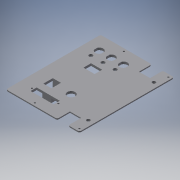
# Autodesk Inventor part: vrch2
Saved by Autodesk Inventor 2016 (Build 200138000, 138)
## iProperties
Created: 2015-11-06
Part Number: vrch2
Material: Generic
Document SubType Name: Modeling
Designer: Jufo
Density: 1 g/cm^3
Appearance: Default
Author: Jufo
Autodesk Inventor part; units mm, degrees
ref_plane "YZ Plane" through (0, 0, 0) normal (1, 0, 0) x (0, 1, 0)
ref_plane "XZ Plane" through (0, 0, 0) normal (0, 1, 0) x (-1, 0, 0)
ref_plane "XY Plane" through (0, 0, 0) normal (0, 0, 1) x (1, 0, 0)
sketch "Sketch1" plane through (0, 0, 0) normal (0, 1, 0) x (-1, 0, 0)
  line L0 (8.278, -23.2242) -> (24.278, -23.2242)
  line L1 (24.278, -23.2242) -> (24.278, 3.7758)
  line L2 (24.278, 3.7758) -> (48.278, 3.7758)
  line L3 (48.278, 3.7758) -> (48.278, -23.2242)
  line L4 (48.278, -23.2242) -> (88.278, -23.2242)
  line L5 (48.278, -23.2242) -> (136.1936, -23.2242)
  line L6 (136.1936, -23.2242) -> (136.1936, 142.7758)
  line L7 (136.1936, 142.7758) -> (48.278, 142.7758)
  line L8 (48.278, 142.7758) -> (48.278, 115.7758)
  line L9 (48.278, 115.7758) -> (24.278, 115.7758)
  line L10 (24.278, 115.7758) -> (24.278, 142.7758)
  line L11 (24.278, 142.7758) -> (24.278, 115.7758)
  line L12 (8.278, 142.7758) -> (24.278, 142.7758)
  line L13 (24.278, 142.7758) -> (8.278, 142.7758)
  line L14 (8.278, 142.7758) -> (8.278, -23.2242)
  line L15 (24.278, 3.7758) -> (24.278, -23.2242)
  circle A0 centre (11.278, -20.2242) radius 1.5
  circle A1 centre (11.278, -20.2242) radius 1.5
  circle A2 centre (11.278, 139.7758) radius 1.5
  circle A3 centre (11.278, 139.7758) radius 1.5
  circle A4 centre (91.278, -20.2242) radius 1.5
  circle A5 centre (91.278, -20.2242) radius 1.5
  circle A6 centre (91.278, 139.7758) radius 1.5
  circle A7 centre (91.278, 139.7758) radius 1.5
  line L16 (133.1936, 141.7758) -> (49.278, 141.7758)
  line L17 (49.278, 141.7758) -> (49.278, 114.7758)
  line L18 (49.278, 114.7758) -> (23.278, 114.7758)
  line L19 (23.278, 114.7758) -> (23.278, 141.7758)
  line L20 (8.278, 59.7758) -> (68.278, 59.7758)
  line L21 (133.1936, 141.7758) -> (133.1936, 59.7758)
  line L22 (23.278, 141.7758) -> (9.278, 141.7758)
  line L23 (9.278, 141.7758) -> (9.278, 59.7758)
  line L24 (133.1936, -22.2242) -> (49.278, -22.2242)
  line L25 (49.278, -22.2242) -> (49.278, 4.7758)
  line L26 (49.278, 4.7758) -> (23.278, 4.7758)
  line L27 (23.278, 4.7758) -> (23.278, -22.2242)
  line L28 (133.1936, -22.2242) -> (133.1936, 59.7758)
  line L29 (23.278, -22.2242) -> (9.278, -22.2242)
  line L30 (9.278, -22.2242) -> (9.278, 59.7758)
  point P0 (0, 0)
  point P1 (0, 0)
  dimension "d0" = 24
  dimension "d1" = 16
  dimension "d2" = 87.9156
  dimension "d3" = 166
  dimension "d4" = 3
  dimension "d5" = 27
  dimension "d6" = 1
  dimension "d8" = 1
  dimension "d9" = 1
  dimension "d10" = 1
  dimension "d11" = 1
  constraints: 62 end point, 13 perpendicular, 8 centre point, 6 symmetric about line, 5 point on line, 4 coincident, 3 horizontal, 2 parallel, 1 midpoint, 1 vertical
  measures "d0" distance of L8.end L9.end
  measures "d1" distance of L10.end L12.start
  measures "d2" distance of L6.end L7.end
  measures "d3" distance of L5.end L6.end
  measures "d4" distance between parallel lines of L6 L21
  measures "d5" distance of L7.end L8.end
  measures "d6" distance between parallel lines of L8 L17
  measures "d8" distance between parallel lines of L18 L9
  measures "d9" distance between parallel lines of L19 L10
  measures "d10" distance between parallel lines of L12 L22
  measures "d11" distance between parallel lines of L14 L23
extrude "Extrusion1" add sketch "Sketch1" along normal blind 2 contours L21 L28 L24 L25 L26 L27 L29 L30 L23 L22 L19 L18 L17 L16
sketch "Sketch2" plane through (0, 2, 0) normal (0, 1, 0) x (1, 0, 0)
  line L0 (-6.278, 25.2242) -> (-26.278, 25.2242)
  line L1 (-26.278, 25.2242) -> (-26.278, 2.2242)
  line L2 (-26.278, 2.2242) -> (-46.278, 2.2242)
  line L3 (-46.278, 2.2242) -> (-46.278, 25.2242)
  line L4 (-46.278, 25.2242) -> (-138.2936, 25.2242)
  line L5 (-133.1936, 22.2242) -> (-133.1936, -141.7758) projected
  line L6 (-133.1936, -59.7758) -> (-63.3349, -59.7758)
  line L7 (-138.2936, 25.2242) -> (-138.2936, -59.7758)
  line L8 (-6.278, 25.2242) -> (-6.278, -59.7758)
  line L9 (-9.278, -141.7758) -> (-9.278, 22.2242) projected
  line L10 (-9.278, 22.2242) -> (-23.278, 22.2242) projected
  line L11 (-23.278, 22.2242) -> (-23.278, -4.7758) projected
  line L12 (-23.278, -4.7758) -> (-49.278, -4.7758) projected
  line L13 (-49.278, -4.7758) -> (-49.278, 22.2242) projected
  line L14 (-49.278, 22.2242) -> (-133.1936, 22.2242) projected
  line L15 (-6.278, -144.7758) -> (-26.278, -144.7758)
  line L16 (-26.278, -144.7758) -> (-26.278, -121.7758)
  line L17 (-26.278, -121.7758) -> (-46.278, -121.7758)
  line L18 (-46.278, -121.7758) -> (-46.278, -144.7758)
  line L19 (-46.278, -144.7758) -> (-138.2936, -144.7758)
  line L20 (-6.278, -144.7758) -> (-6.278, -59.7758)
  line L21 (-138.2936, 25.2242) -> (-138.2936, -144.7758)
  circle A0 centre (-91.278, 20.2242) radius 1.5 projected
  circle A1 centre (-91.278, 20.2242) radius 1.5
  circle A2 centre (-91.278, -139.7758) radius 1.5 projected
  circle A3 centre (-91.278, -139.7758) radius 1.5
  circle A4 centre (-11.278, -139.7758) radius 1.5 projected
  circle A5 centre (-11.278, -139.7758) radius 1.5
  circle A6 centre (-11.278, 20.2242) radius 1.5
  point P0 (0, 0)
  dimension "d14" = 3
  dimension "d15" = 3
  dimension "d16" = 3
  dimension "d17" = 7
  dimension "d18" = 3
  dimension "d19" = 3
  dimension "d130" = 5.1
  constraints: 30 end point, 6 symmetric about line, 5 point on line, 4 centre point, 4 perpendicular, 3 coincident, 2 horizontal, 1 concentric, 1 midpoint, 1 parallel, 1 vertical
  measures "d14" distance between parallel lines of L8 L9
  measures "d15" distance between parallel lines of L0 L10
  measures "d16" distance between parallel lines of L1 L11
  measures "d17" distance between parallel lines of L12 L2
  measures "d18" distance between parallel lines of L13 L3
  measures "d19" distance between parallel lines of L4 L14
  measures "d130" distance between parallel lines of L5 L21
extrude "Extrusion2" add sketch "Sketch2" along normal blind 2
sketch "Sketch9" plane through (0, 4, 0) normal (0, 1, 0) x (1, 0, 0)
  line L0 (-26.278, -121.7758) -> (-6.278, -121.7758)
  line L1 (-6.278, -144.7758) -> (-6.278, 25.2242) projected
  line L2 (-26.278, 2.2242) -> (-6.278, 2.2242)
  line L3 (-16.278, -121.7758) -> (-16.278, -118.7758)
  circle A0 centre (-16.278, -118.7758) radius 3
  line L4 (-16.278, 2.2242) -> (-16.278, -0.7758)
  circle A1 centre (-16.278, -0.7758) radius 3
  line L5 (-102.439, -41.2758) -> (-82.439, -41.2758)
  line L6 (-82.439, -41.2758) -> (-82.439, -27.7758)
  line L7 (-82.439, -27.7758) -> (-102.439, -27.7758)
  line L8 (-102.439, -27.7758) -> (-102.439, -41.2758)
  line L9 (-26.278, 2.2242) -> (-46.278, 2.2242) projected
  line L10 (-26.278, 25.2242) -> (-26.278, 2.2242) projected
  line L11 (-113.628, -102.2758) -> (-99.128, -102.2758)
  line L12 (-99.128, -102.2758) -> (-99.128, -85.2758)
  line L13 (-99.128, -85.2758) -> (-113.628, -85.2758)
  line L14 (-113.628, -85.2758) -> (-113.628, -102.2758)
  circle A2 centre (-72.128, -93.7758) radius 7
  circle A3 centre (-114.678, -0.7758) radius 7
  circle A4 centre (-92.878, -0.7758) radius 7
  circle A5 centre (-71.078, -0.7758) radius 7
  line L15 (-121.6758, -0.6001) -> (-121.6758, -0.6001)
  line L16 (-99.8758, -0.9515) -> (-99.8758, -0.6001)
  circle A6 centre (-114.678, -15.7758) radius 3.25
  circle A7 centre (-92.878, -15.7758) radius 3.25
  circle A8 centre (-71.078, -15.7758) radius 3.25
  line L17 (-46.278, 25.2242) -> (-138.2936, 25.2242) projected
  line L18 (-49.278, -4.7758) -> (-49.278, 22.2242) projected
  line L19 (-138.2936, 25.2242) -> (-138.2936, -144.7758) projected
  line L20 (-113.628, -125.2758) -> (-72.128, -125.2758)
  line L21 (-72.128, -125.2758) -> (-72.128, -114.2758)
  line L22 (-72.128, -114.2758) -> (-113.628, -114.2758)
  line L23 (-113.628, -114.2758) -> (-113.628, -125.2758)
  line L24 (-46.278, -121.7758) -> (-26.278, -121.7758) projected
  line L25 (-113.628, -119.7758) -> (-116.628, -119.7758)
  circle A9 centre (-116.628, -119.7758) radius 1.5
  line L26 (-72.128, -119.7758) -> (-69.128, -119.7758)
  circle A10 centre (-69.128, -119.7758) radius 1.5
  line L27 (-99.0879, -4.0066) -> (-99.0879, 2.455)
  line L28 (-120.8879, -4.0066) -> (-120.8879, 2.455)
  line L29 (-77.2879, -4.0066) -> (-77.2879, 2.455)
  line L30 (-46.278, -144.7758) -> (-46.278, -121.7758) projected
  line L31 (-64.8682, 2.455) -> (-64.8682, -4.0066)
  line L32 (-86.6682, 2.455) -> (-86.6682, -4.0066)
  line L33 (-108.4682, 2.455) -> (-108.4682, -4.0066)
  arc A11 (-108.4682, -4.0066) -> (-108.4682, 2.455) centre (-114.678, -0.7758) ccw
  point P0 (0, 0)
  dimension "d62" = 3
  dimension "d63" = 6
  dimension "d64" = 3
  dimension "d65" = 13.5
  dimension "d66" = 20
  dimension "d67" = 30
  dimension "d69" = 20
  dimension "d70" = 17
  dimension "d71" = 14.5
  dimension "d72" = 14
  dimension "d75" = 14
  dimension "d76" = 14
  dimension "d77" = 14
  dimension "d78" = 21.8
  dimension "d79" = 21.8
  dimension "d80" = 6.5
  dimension "d81" = 6.5
  dimension "d82" = 6.5
  dimension "d83" = 15
  dimension "d84" = 15
  dimension "d85" = 15
  dimension "d89" = 21.8
  dimension "d90" = 21.8
  dimension "d92" = 21.8
  dimension "d93" = 21.8
  dimension "d97" = 11
  dimension "d98" = 41.5
  dimension "d99" = 7.5
  dimension "d100" = 3
  dimension "d101" = 3
  dimension "d102" = 3
  dimension "d103" = 3
  dimension "d106" = 25.85
  dimension "d108" = 0
  dimension "d109" = 20.5
  constraints: 52 end point, 18 point on circle, 12 centre point, 10 parallel, 7 vertical, 6 horizontal, 4 coincident, 4 midpoint, 3 perpendicular, 2 point on line, 1 concentric, 1 tangent
  measures "d62" distance of L3.start L3.end
  measures "d63" diameter of A0
  measures "d64" distance of L4.start L4.end
  measures "d65" distance of L5.end L6.end
  measures "d66" distance of L6.end L7.end
  measures "d67" distance between parallel lines of L9 L7
  measures "d69" distance between parallel lines of L1 L10
  measures "d70" distance of L11.end L12.end
  measures "d71" distance of L12.end L13.end
  measures "d72" diameter of A2
  measures "d75" diameter of A3
  measures "d76" diameter of A4
  measures "d77" diameter of A5
  measures "d78" distance of A4.centre A3.centre
  measures "d79" distance of A5.centre A4.centre
  measures "d80" diameter of A6
  measures "d81" diameter of A7
  measures "d82" diameter of A8
  measures "d83" distance of A6.centre A3.centre
  measures "d84" distance of A4.centre A7.centre
  measures "d85" distance of A5.centre A8.centre
  measures "d89" distance of A7.centre A8.centre
  measures "d90" distance of A7.centre A6.centre
  measures "d92" distance from line of L18 A8.centre
  measures "d93" distance from line of L18 A5.centre
  measures "d97" distance of L20.end L21.end
  measures "d98" distance of L21.end L22.end
  measures "d99" distance between parallel lines of L22 L24
  measures "d100" distance of L25.start L25.end
  measures "d101" diameter of A9
  measures "d102" distance of L26.start L26.end
  measures "d103" diameter of A10
  measures "d106" distance between parallel lines of L30 L21
  measures "d108" distance between parallel lines of L23 L14
  measures "d109" distance from line of A2.centre L22
extrude "Extrusion8" cut sketch "Sketch9" against normal blind 15 contours A0 | A1 | L8 L7 L6 L5 | L14 L13 L12 L11 | A2 | L33 A3 L28 | L32 A4 L27 | L31 A5 L29 | A6 | A7 | A8 | L23 L22 L21 L20 | A9 | A10
fillet "Fillet1" radius 3 8 edges at (-46.278, 3, -25.2242) (-26.278, 3, -25.2242) (-6.278, 3, -25.2242) (-6.278, 3, 144.7758) (-46.278, 3, 144.7758) (-26.278, 3, 144.7758) (-138.2936, 3, -25.2242) (-138.2936, 3, 144.7758)
sketch "Sketch10" plane through (0, 0, 0) normal (0, -1, 0) x (1, 0, 0)
  line L0 (-113.628, 85.2758) -> (-113.628, 83.2758)
  line L1 (-113.628, 83.2758) -> (-97.128, 83.2758)
  line L2 (-97.128, 83.2758) -> (-97.128, 104.2758)
  line L3 (-97.128, 104.2758) -> (-113.628, 104.2758)
  line L4 (-113.628, 104.2758) -> (-113.628, 102.2758)
  line L5 (-99.128, 102.2758) -> (-99.128, 85.2758) projected
  line L6 (-113.628, 102.2758) -> (-99.128, 102.2758) projected
  line L7 (-113.628, 85.2758) -> (-99.128, 85.2758)
  line L8 (-99.128, 85.2758) -> (-99.128, 102.2758)
  line L9 (-99.128, 102.2758) -> (-113.628, 102.2758)
  point P0 (0, 0)
  dimension "d112" = 2
  dimension "d113" = 2
  dimension "d114" = 2
  constraints: 16 end point, 5 perpendicular, 1 collinear, 1 horizontal, 1 point on line, 1 vertical
  measures "d112" distance of L0.start L0.end
  measures "d113" distance between parallel lines of L2 L5
  measures "d114" distance between parallel lines of L3 L6
extrude "Extrusion9" add sketch "Sketch10" along normal blind 17
sketch "Sketch11" plane through (0, 0, 0) normal (0, -1, 0) x (1, 0, 0)
  circle A0 centre (-72.128, 93.7758) radius 7 projected
  line L0 (-69.8349, 79.8078) -> (-67.8349, 79.8078)
  line L1 (-67.8349, 79.8078) -> (-67.8349, 84.7028)
  line L2 (-67.8349, 84.7028) -> (-69.8349, 84.7028)
  line L3 (-71.4349, 84.7028) -> (-71.4349, 79.8078)
  line L4 (-71.4349, 79.8078) -> (-73.4349, 79.8078)
  line L5 (-73.4349, 79.8078) -> (-73.4349, 84.7028)
  line L6 (-73.4349, 84.7028) -> (-71.4349, 84.7028)
  line L7 (-69.8349, 84.7028) -> (-69.8349, 79.8078)
  line L8 (-70.6349, 85.8044) -> (-70.6349, 78.1264)
  point P0 (0, 0)
  dimension "d117" = 2
  dimension "d118" = 2
  dimension "d120" = 0.8
  dimension "d121" = 0.8
  constraints: 18 end point, 5 perpendicular, 4 point on line, 2 vertical, 1 horizontal
  measures "d117" distance of L1.end L2.end
  measures "d118" distance of L5.end L3.start
  measures "d120" distance between parallel lines of L7 L8
  measures "d121" distance between parallel lines of L8 L3
extrude "Extrusion10" add sketch "Sketch11" along normal blind 8 contours L7 L2 L1 L0 | L3 L4 L5 L6
sketch "Sketch12" plane through (-67.8349, 0, 84.7028) normal (1, 0, 0) x (0, 0, -1)
  circle A0 centre (1.695, -6.5) radius 1
  line L0 (4.895, 0) -> (4.895, -8) projected
  line L1 (4.895, -8) -> (0, -8) projected
  point P0 (84.7028, 0)
  point P1 (0, 0)
  dimension "d124" = 2
  dimension "d126" = 3.2
  dimension "d127" = 1.5
  constraints: 1 centre point
  measures "d124" diameter of A0
  measures "d126" distance from line of L0 A0.centre
  measures "d127" distance from line of L1 A0.centre
extrude "Extrusion11" cut sketch "Sketch12" against normal blind 8
sketch "Sketch15" plane through (0, 2, 0) normal (0, -1, 0) x (1, 0, 0)
  line L0 (-138.2936, -25.2242) -> (-138.2936, 144.7758) projected
  line L1 (-138.2936, 4.7758) -> (-133.1361, 4.7758)
  line L2 (-138.2936, 114.7758) -> (-133.1361, 114.7758)
  line L3 (-133.1361, 114.7758) -> (-133.1361, 4.7758)
  line L4 (-138.2936, 4.7758) -> (-138.2936, 114.7758)
  line L5 (-49.278, -25.2242) -> (-138.2936, -25.2242) projected
  point P0 (0, 0)
  dimension "d131" = 110
  dimension "d132" = 30
  constraints: 8 end point, 2 horizontal, 2 point on line, 1 collinear, 1 perpendicular
  measures "d131" distance between parallel lines of L1 L2
  measures "d132" distance between parallel lines of L1 L5
extrude "Extrusion12" add sketch "Sketch15" along normal blind 2
equation "\"d78\" = d92"
equation "\"d79\" = d92"
equation "\"d89\" = d92"
equation "\"d90\" = d92"
equation "\"d93\" = d79"
equation "\"d104\" = d85"
body "Solid1"
